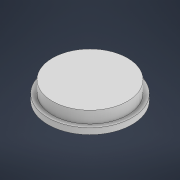
# Autodesk Inventor part: InputShaft2
Saved by Autodesk Inventor 2021 (Build 250183000, 183)
## iProperties
Created: 2022-10-09
Part Number: InputShaft2
Material: Ogólny
Document SubType Name: Modeling
Designer: MicnedSQ
Density: 1 g/cm^3
Appearance: Domyślna
Author: MicnedSQ
Autodesk Inventor part; units mm, degrees
ref_plane "YZ Plane" through (0, 0, 0) normal (1, 0, 0) x (0, 1, 0)
ref_plane "XZ Plane" through (0, 0, 0) normal (0, 1, 0) x (-1, 0, 0)
ref_plane "XY Plane" through (0, 0, 0) normal (0, 0, 1) x (1, 0, 0)
sketch "Szkic1" plane through (0, 0, 0) normal (0, 1, 0) x (-1, 0, 0)
  circle A0 centre (0, 0) radius 14
  dimension "d0" = 28
  constraints: 1 centre point, 1 coincident
  measures "d0" diameter of A0
extrude "Wyciągnięcie proste1" add sketch "Szkic1" along normal blind 2
sketch "Szkic2" plane through (0, 2, 0) normal (0, 1, 0) x (1, 0, 0)
  circle A0 centre (0, 0) radius 12.5
  dimension "d3" = 25
  constraints: 1 centre point, 1 coincident
  measures "d3" diameter of A0
extrude "Wyciągnięcie proste2" add sketch "Szkic2" along normal blind 4
